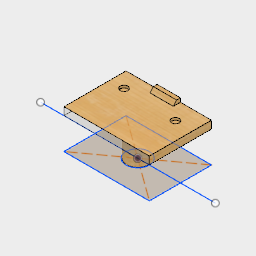
tavolo v4 (Autodesk Fusion 360 design; units mm, degrees)
Autodesk Fusion 360 part; units mm, degrees
sketch "Sketch1" plane through (0, 0, 0) normal (0, 1, 0) x (1, 0, 0)
  line L0 (-125, 0) -> (100, 0)
  circle A0 centre (0, 0) radius 15
  line L1 (-55, 40) -> (55, 40)
  line L2 (55, 40) -> (55, -40)
  line L3 (55, -40) -> (-55, -40)
  line L4 (-55, -40) -> (-55, 40)
  line L5 (-55, 40) -> (55, -40) construction
  line L6 (55, 40) -> (-55, -40) construction
cylinder "CylinderPrimitive1" add diameter 29.045 height 40 placed x (1, 0, 0) y (0, 0, -1) z (0, 1, 0) at (0, 0, 0)
form "Form1" [no effect]
ref_plane "WorkPlane1" through (0, 40, 0) normal (0, 1, 0) x (1, 0, 0)
box "BoxPrimitive1" add length 80 width 110 height 10 placed x (0, 0, 1) y (1, 0, 0) z (0, 1, 0) at (-55, 40, -40)
hole "Hole1" at (-36.7157, 50, -19.1237) direction (0, -1, 0) diameter 10 depth 3 tip angle 118
hole "Hole2" at (32.3628, 50, -16.1913) direction (0, -1, 0) diameter 10 depth 3 tip angle 118
ref_plane "WorkPlane2" through (0, 50, 0) normal (0, 1, 0) x (0, 0, 1)
box "BoxPrimitive2" add length 5 width 30 height 5 placed x (0, 0, 1) y (1, 0, 0) z (0, 1, 0) at (-15, 50, -40)
draft "Draft1" angle 40 neutral plane through (-15, 55, -40) pull (0, 1, 0) 1 faces at (-5, 51.6667, -35)
